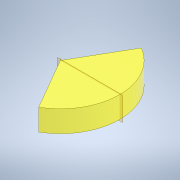
# Autodesk Inventor part: largeCap
Saved by Autodesk Inventor 2021.1 (Build 251245000, 245)
## iProperties
Created: 2020-09-25
Part Number: largeCap
Material: PC/ABS Plastic
Document SubType Name: Modeling
Designer: robst
Density: 0.357273 g/cm^3
Appearance: Smooth - Yellow
Author: robst
Autodesk Inventor part; units mm, degrees
ref_plane "XZ Plane" through (0, 0, 0) normal (0, 1, 0) x (-1, 0, 0)
sketch "Sketch1" plane through (0, 0, 0) normal (0, 0, 1) x (1, 0, 0)
  line L0 (0, 0) -> (122.2375, 0)
  line L1 (122.2375, 0) -> (122.2375, -44.45)
  line L2 (122.2375, -44.45) -> (115.8875, -44.45)
  line L3 (115.8875, -44.45) -> (115.8875, -6.35)
  line L4 (115.8875, -6.35) -> (0, -6.35)
  line L5 (0, -6.35) -> (0, 0)
  dimension "d2" = 6.35
  dimension "d3" = 6.35
  dimension "d4" = 115.8875
  dimension "d5" = 38.1
  constraints: 12 end point, 4 perpendicular, 1 horizontal, 1 parallel
  measures "d2" distance between parallel lines of L4 L0
  measures "d3" distance between parallel lines of L1 L3
  measures "d4" distance from line of L3 L0.start
  measures "d5" distance from line of L2.end L4
revolve "Revolution1" add sketch "Sketch1" angle 120 mid plane about axis through (0, -6.35, 0) along (0, 1, 0)
ref_plane "Work Plane1" through (57.9438, -44.45, -100.3615) normal (1, 0, 0) x (0, 1, 0)
sketch "Sketch7" plane through (57.9438, -44.45, -100.3615) normal (1, 0, 0) x (0, 1, 0)
  line L0 (38.1, 0) -> (38.1, 100.3615) projected
  line L1 (44.45, 100.3615) -> (38.1, 100.3615) projected
  line L2 (44.45, 100.3615) -> (44.45, -5.4993) projected
  line L3 (44.45, -5.4993) -> (0, -5.4993) projected
  line L4 (0, -5.4993) -> (0, 0) projected
  line L5 (0, 0) -> (38.1, 0) projected
  line L6 (38.1, 0) -> (38.1, 200.723) projected
  line L7 (38.1, 100.3615) -> (38.1, 200.723) projected
  line L8 (38.1, 200.723) -> (0, 200.723) projected
  line L9 (0, 200.723) -> (0, 206.2223) projected
  line L10 (0, 206.2223) -> (44.45, 206.2223) projected
  line L11 (44.45, 206.2223) -> (44.45, 100.3615) projected
  line L12 (44.45, 100.3615) -> (38.1, 100.3615) projected
  line L13 (19.05, 0) -> (19.05, 200.723) construction
  line L14 (15.24, 56.8306) -> (15.24, 52.4154)
  line L15 (15.24, 52.4154) -> (22.86, 52.4154)
  line L16 (22.86, 52.4154) -> (22.86, 53.4281)
  line L17 (22.86, 53.4281) -> (16.1416, 53.4281)
  line L18 (16.1416, 53.4281) -> (16.1416, 56.8306)
  line L19 (16.1416, 56.8306) -> (15.24, 56.8306)
  spline S0 degree 2 poles (15.8452, 60.7394) (15.7587, 60.622) (15.45, 60.2268) (15.3573, 60.0416) knots 0 0 0 1 2 2 2
  spline S1 degree 2 poles (15.3573, 60.0416) (15.2215, 59.7884) (15.0794, 59.3129) (15.0794, 58.8807) knots 0 0 0 1 2 2 2
  spline S2 degree 2 poles (15.0794, 58.8807) (15.0794, 58.5287) (15.345, 57.8927) (15.5858, 57.6518) knots 0 0 0 1 2 2 2
  spline S3 degree 2 poles (15.5858, 57.6518) (15.8205, 57.4234) (16.5121, 57.1455) (16.8949, 57.1455) knots 0 0 0 1 2 2 2
  spline S4 degree 2 poles (16.8949, 57.1455) (17.4877, 57.1455) (18.3275, 57.6457) (18.5683, 58.1891) knots 0 0 0 1 2 2 2
  spline S5 degree 2 poles (18.5683, 58.1891) (18.7906, 58.6707) (18.9574, 59.9798) (19.0006, 60.7394) knots 0 0 0 1 2 2 2
  line L20 (19.0006, 60.7394) -> (19.1859, 60.7394)
  spline S6 degree 2 poles (19.1859, 60.7394) (19.5193, 60.7394) (19.933, 60.5356) (20.0504, 60.3503) knots 0 0 0 1 2 2 2
  spline S7 degree 2 poles (20.0504, 60.3503) (20.1677, 60.1651) (20.2418, 59.634) (20.2418, 59.35) knots 0 0 0 1 2 2 2
  spline S8 degree 2 poles (20.2418, 59.35) (20.2418, 59.0165) (20.0442, 58.115) (19.8528, 57.6642) knots 0 0 0 1 2 2 2
  line L21 (19.8528, 57.6642) -> (19.8528, 57.6086)
  line L22 (19.8528, 57.6086) -> (20.8346, 57.6086)
  spline S9 degree 2 poles (20.8346, 57.6086) (20.9087, 57.8741) (21.0939, 58.8683) (21.0939, 59.3562) knots 0 0 0 1 2 2 2
  spline S10 degree 2 poles (21.0939, 59.3562) (21.0939, 59.949) (20.9087, 60.7579) (20.6679, 61.079) knots 0 0 0 1 2 2 2
  spline S11 degree 2 poles (20.6679, 61.079) (20.4332, 61.3939) (19.686, 61.7027) (19.1488, 61.7027) knots 0 0 0 1 2 2 2
  line L23 (19.1488, 61.7027) -> (15.24, 61.7027)
  line L24 (15.24, 61.7027) -> (15.24, 60.7394)
  line L25 (15.24, 60.7394) -> (15.8452, 60.7394)
  line L26 (16.6479, 60.7394) -> (18.2349, 60.7394)
  spline S12 degree 2 poles (18.2349, 60.7394) (18.204, 60.3936) (18.099, 59.35) (18.0002, 59.0227) knots 0 0 0 1 2 2 2
  spline S13 degree 2 poles (18.0002, 59.0227) (17.8829, 58.6399) (17.3951, 58.1397) (16.9628, 58.1397) knots 0 0 0 1 2 2 2
  spline S14 degree 2 poles (16.9628, 58.1397) (16.4688, 58.1397) (15.9687, 58.6954) (15.9687, 59.2265) knots 0 0 0 1 2 2 2
  spline S15 degree 2 poles (15.9687, 59.2265) (15.9687, 59.6773) (16.3577, 60.4183) (16.6479, 60.7394) knots 0 0 0 1 2 2 2
  line L27 (19.9269, 66.087) -> (19.9269, 66.0376)
  spline S16 degree 2 poles (19.9269, 66.0376) (19.9577, 65.9264) (19.9701, 65.6856) (19.9701, 65.5188) knots 0 0 0 1 2 2 2
  spline S17 degree 2 poles (19.9701, 65.5188) (19.9701, 65.1298) (19.6305, 64.3641) (19.297, 64.0183) knots 0 0 0 1 2 2 2
  line L28 (19.297, 64.0183) -> (15.24, 64.0183)
  line L29 (15.24, 64.0183) -> (15.24, 63.055)
  line L30 (15.24, 63.055) -> (20.9581, 63.055)
  line L31 (20.9581, 63.055) -> (20.9581, 64.0183)
  line L32 (20.9581, 64.0183) -> (20.1059, 64.0183)
  spline S18 degree 2 poles (20.1059, 64.0183) (20.5752, 64.5432) (20.9581, 65.3274) (20.9581, 65.6979) knots 0 0 0 1 2 2 2
  spline S19 degree 2 poles (20.9581, 65.6979) (20.9581, 65.8461) (20.9457, 65.9943) (20.9272, 66.087) knots 0 0 0 1 2 2 2
  line L33 (20.9272, 66.087) -> (19.9269, 66.087)
  spline S20 degree 2 poles (14.3261, 67.0379) (14.2829, 67.1367) (14.147, 67.5134) (14.0914, 67.7542) knots 0 0 0 1 2 2 2
  spline S21 degree 2 poles (14.0914, 67.7542) (14.0235, 68.0197) (13.9432, 68.4705) (13.9432, 68.736) knots 0 0 0 1 2 2 2
  spline S22 degree 2 poles (13.9432, 68.736) (13.9432, 69.1806) (14.1779, 69.7982) (14.3878, 69.9711) knots 0 0 0 1 2 2 2
  spline S23 degree 2 poles (14.3878, 69.9711) (14.5978, 70.1378) (15.1474, 70.2675) (15.4994, 70.2675) knots 0 0 0 1 2 2 2
  line L34 (15.4994, 70.2675) -> (15.9995, 70.2675)
  spline S24 degree 2 poles (15.9995, 70.2675) (15.6599, 69.8784) (15.3388, 69.1312) (15.3388, 68.5693) knots 0 0 0 1 2 2 2
  spline S25 degree 2 poles (15.3388, 68.5693) (15.3388, 67.5937) (16.7899, 66.4389) (18.1546, 66.4389) knots 0 0 0 1 2 2 2
  spline S26 degree 2 poles (18.1546, 66.4389) (18.8647, 66.4389) (19.9639, 66.8403) (20.3529, 67.1738) knots 0 0 0 1 2 2 2
  spline S27 degree 2 poles (20.3529, 67.1738) (20.7173, 67.4949) (21.1186, 68.3779) (21.1186, 68.8472) knots 0 0 0 1 2 2 2
  spline S28 degree 2 poles (21.1186, 68.8472) (21.1186, 69.2918) (20.9087, 69.9402) (20.7173, 70.2675) knots 0 0 0 1 2 2 2
  line L35 (20.7173, 70.2675) -> (20.9581, 70.323)
  line L36 (20.9581, 70.323) -> (20.9581, 71.2308)
  line L37 (20.9581, 71.2308) -> (15.8946, 71.2308)
  spline S29 degree 2 poles (15.8946, 71.2308) (14.4372, 71.2308) (13.0787, 69.9649) (13.0787, 68.6619) knots 0 0 0 1 2 2 2
  spline S30 degree 2 poles (13.0787, 68.6619) (13.0787, 68.242) (13.2146, 67.3652) (13.3257, 66.9885) knots 0 0 0 1 2 2 2
  line L38 (13.3257, 66.9885) -> (14.3261, 66.9885)
  line L39 (14.3261, 66.9885) -> (14.3261, 67.0379)
  line L40 (16.7899, 70.2675) -> (19.933, 70.2675)
  spline S31 degree 2 poles (19.933, 70.2675) (20.1059, 69.9093) (20.2541, 69.3041) (20.2541, 69.0016) knots 0 0 0 1 2 2 2
  spline S32 degree 2 poles (20.2541, 69.0016) (20.2541, 68.2729) (19.1797, 67.4331) (18.1731, 67.4331) knots 0 0 0 1 2 2 2
  spline S33 degree 2 poles (18.1731, 67.4331) (17.2222, 67.4331) (16.228, 68.0691) (16.228, 68.7854) knots 0 0 0 1 2 2 2
  spline S34 degree 2 poles (16.228, 68.7854) (16.228, 69.1621) (16.5244, 69.9525) (16.7899, 70.2675) knots 0 0 0 1 2 2 2
  spline S35 degree 2 poles (15.1103, 75.1087) (15.1103, 73.7378) (16.6479, 72.2311) (18.0682, 72.2311) knots 0 0 0 1 2 2 2
  spline S36 degree 2 poles (18.0682, 72.2311) (19.4637, 72.2311) (21.1186, 73.6946) (21.1186, 74.874) knots 0 0 0 1 2 2 2
  spline S37 degree 2 poles (21.1186, 74.874) (21.1186, 75.4051) (20.8099, 76.2264) (20.4826, 76.5289) knots 0 0 0 1 2 2 2
  spline S38 degree 2 poles (20.4826, 76.5289) (20.1553, 76.8377) (19.2106, 77.165) (18.5251, 77.165) knots 0 0 0 1 2 2 2
  line L41 (18.5251, 77.165) -> (18.0002, 77.165)
  line L42 (18.0002, 77.165) -> (18.0002, 73.2068)
  spline S39 degree 2 poles (18.0002, 73.2068) (17.0061, 73.2068) (15.9501, 74.2071) (15.9501, 75.0963) knots 0 0 0 1 2 2 2
  spline S40 degree 2 poles (15.9501, 75.0963) (15.9501, 75.4113) (16.0922, 76.0226) (16.2033, 76.2696) knots 0 0 0 1 2 2 2
  spline S41 degree 2 poles (16.2033, 76.2696) (16.3268, 76.5289) (16.5429, 76.8871) (16.6417, 77.0044) knots 0 0 0 1 2 2 2
  line L43 (16.6417, 77.0044) -> (16.6417, 77.06)
  line L44 (16.6417, 77.06) -> (15.592, 77.06)
  spline S42 degree 2 poles (15.592, 77.06) (15.5241, 76.8933) (15.3265, 76.3869) (15.2709, 76.1893) knots 0 0 0 1 2 2 2
  spline S43 degree 2 poles (15.2709, 76.1893) (15.1906, 75.9114) (15.1103, 75.4545) (15.1103, 75.1087) knots 0 0 0 1 2 2 2
  spline S44 degree 2 poles (18.7351, 76.2264) (19.1241, 76.214) (19.6922, 76.0535) (19.8836, 75.8991) knots 0 0 0 1 2 2 2
  spline S45 degree 2 poles (19.8836, 75.8991) (20.0998, 75.7324) (20.3282, 75.2075) (20.3282, 74.8185) knots 0 0 0 1 2 2 2
  spline S46 degree 2 poles (20.3282, 74.8185) (20.3282, 74.4356) (20.0998, 73.8984) (19.8775, 73.6761) knots 0 0 0 1 2 2 2
  spline S47 degree 2 poles (19.8775, 73.6761) (19.649, 73.46) (19.0994, 73.2377) (18.7351, 73.2068) knots 0 0 0 1 2 2 2
  line L45 (18.7351, 73.2068) -> (18.7351, 76.2264)
  spline S48 degree 2 poles (15.1041, 84.4639) (15.1041, 83.7229) (15.6043, 82.4693) (16.1045, 82.0124) knots 0 0 0 1 2 2 2
  spline S49 degree 2 poles (16.1045, 82.0124) (16.5985, 81.5554) (18.0805, 81.0553) (19.0438, 81.0553) knots 0 0 0 1 2 2 2
  spline S50 degree 2 poles (19.0438, 81.0553) (20.001, 81.0553) (21.4212, 81.5431) (21.9461, 82.0062) knots 0 0 0 1 2 2 2
  spline S51 degree 2 poles (21.9461, 82.0062) (22.4586, 82.4632) (22.9959, 83.7105) (22.9959, 84.4824) knots 0 0 0 1 2 2 2
  spline S52 degree 2 poles (22.9959, 84.4824) (22.9959, 84.8653) (22.8847, 85.5383) (22.7982, 85.8224) knots 0 0 0 1 2 2 2
  spline S53 degree 2 poles (22.7982, 85.8224) (22.718, 86.0694) (22.4895, 86.5819) (22.3536, 86.8351) knots 0 0 0 1 2 2 2
  line L46 (22.3536, 86.8351) -> (21.131, 86.8351)
  line L47 (21.131, 86.8351) -> (21.131, 86.7548)
  spline S54 degree 2 poles (21.131, 86.7548) (21.2545, 86.619) (21.6003, 86.1991) (21.767, 85.8965) knots 0 0 0 1 2 2 2
  spline S55 degree 2 poles (21.767, 85.8965) (21.9276, 85.6063) (22.1313, 84.9208) (22.1313, 84.4762) knots 0 0 0 1 2 2 2
  spline S56 degree 2 poles (22.1313, 84.4762) (22.1313, 83.9884) (21.73, 83.1177) (21.3471, 82.7904) knots 0 0 0 1 2 2 2
  spline S57 degree 2 poles (21.3471, 82.7904) (20.9581, 82.4693) (19.7787, 82.1112) (19.0438, 82.1112) knots 0 0 0 1 2 2 2
  spline S58 degree 2 poles (19.0438, 82.1112) (18.2596, 82.1112) (17.1296, 82.4879) (16.7405, 82.8151) knots 0 0 0 1 2 2 2
  spline S59 degree 2 poles (16.7405, 82.8151) (16.3639, 83.1362) (15.981, 83.9946) (15.981, 84.4762) knots 0 0 0 1 2 2 2
  spline S60 degree 2 poles (15.981, 84.4762) (15.981, 84.9147) (16.1971, 85.6618) (16.3577, 85.9521) knots 0 0 0 1 2 2 2
  spline S61 degree 2 poles (16.3577, 85.9521) (16.5182, 86.2299) (16.8517, 86.6437) (16.969, 86.761) knots 0 0 0 1 2 2 2
  line L48 (16.969, 86.761) -> (16.969, 86.8351)
  line L49 (16.969, 86.8351) -> (15.7587, 86.8351)
  spline S62 degree 2 poles (15.7587, 86.8351) (15.6414, 86.5819) (15.4253, 86.1373) (15.3265, 85.8224) knots 0 0 0 1 2 2 2
  spline S63 degree 2 poles (15.3265, 85.8224) (15.2153, 85.4889) (15.1041, 84.9208) (15.1041, 84.4639) knots 0 0 0 1 2 2 2
  spline S64 degree 2 poles (15.8452, 90.8921) (15.7587, 90.7748) (15.45, 90.3796) (15.3573, 90.1943) knots 0 0 0 1 2 2 2
  spline S65 degree 2 poles (15.3573, 90.1943) (15.2215, 89.9411) (15.0794, 89.4657) (15.0794, 89.0334) knots 0 0 0 1 2 2 2
  spline S66 degree 2 poles (15.0794, 89.0334) (15.0794, 88.6814) (15.345, 88.0454) (15.5858, 87.8046) knots 0 0 0 1 2 2 2
  spline S67 degree 2 poles (15.5858, 87.8046) (15.8205, 87.5761) (16.5121, 87.2982) (16.8949, 87.2982) knots 0 0 0 1 2 2 2
  spline S68 degree 2 poles (16.8949, 87.2982) (17.4877, 87.2982) (18.3275, 87.7984) (18.5683, 88.3418) knots 0 0 0 1 2 2 2
  spline S69 degree 2 poles (18.5683, 88.3418) (18.7906, 88.8235) (18.9574, 90.1326) (19.0006, 90.8921) knots 0 0 0 1 2 2 2
  line L50 (19.0006, 90.8921) -> (19.1859, 90.8921)
  spline S70 degree 2 poles (19.1859, 90.8921) (19.5193, 90.8921) (19.933, 90.6883) (20.0504, 90.5031) knots 0 0 0 1 2 2 2
  spline S71 degree 2 poles (20.0504, 90.5031) (20.1677, 90.3178) (20.2418, 89.7868) (20.2418, 89.5027) knots 0 0 0 1 2 2 2
  spline S72 degree 2 poles (20.2418, 89.5027) (20.2418, 89.1693) (20.0442, 88.2677) (19.8528, 87.8169) knots 0 0 0 1 2 2 2
  line L51 (19.8528, 87.8169) -> (19.8528, 87.7613)
  line L52 (19.8528, 87.7613) -> (20.8346, 87.7613)
  spline S73 degree 2 poles (20.8346, 87.7613) (20.9087, 88.0269) (21.0939, 89.0211) (21.0939, 89.5089) knots 0 0 0 1 2 2 2
  spline S74 degree 2 poles (21.0939, 89.5089) (21.0939, 90.1017) (20.9087, 90.9106) (20.6679, 91.2317) knots 0 0 0 1 2 2 2
  spline S75 degree 2 poles (20.6679, 91.2317) (20.4332, 91.5466) (19.686, 91.8554) (19.1488, 91.8554) knots 0 0 0 1 2 2 2
  line L53 (19.1488, 91.8554) -> (15.24, 91.8554)
  line L54 (15.24, 91.8554) -> (15.24, 90.8921)
  line L55 (15.24, 90.8921) -> (15.8452, 90.8921)
  line L56 (16.6479, 90.8921) -> (18.2349, 90.8921)
  spline S76 degree 2 poles (18.2349, 90.8921) (18.204, 90.5463) (18.099, 89.5027) (18.0002, 89.1754) knots 0 0 0 1 2 2 2
  spline S77 degree 2 poles (18.0002, 89.1754) (17.8829, 88.7926) (17.3951, 88.2924) (16.9628, 88.2924) knots 0 0 0 1 2 2 2
  spline S78 degree 2 poles (16.9628, 88.2924) (16.4688, 88.2924) (15.9687, 88.8482) (15.9687, 89.3792) knots 0 0 0 1 2 2 2
  spline S79 degree 2 poles (15.9687, 89.3792) (15.9687, 89.83) (16.3577, 90.571) (16.6479, 90.8921) knots 0 0 0 1 2 2 2
  spline S80 degree 2 poles (18.2534, 97.9996) (16.8208, 97.9996) (15.1288, 96.6349) (15.1288, 95.5913) knots 0 0 0 1 2 2 2
  spline S81 degree 2 poles (15.1288, 95.5913) (15.1288, 95.1652) (15.3265, 94.5107) (15.5302, 94.171) knots 0 0 0 1 2 2 2
  line L57 (15.5302, 94.171) -> (13.1343, 94.171)
  line L58 (13.1343, 94.171) -> (13.1343, 93.2077)
  line L59 (13.1343, 93.2077) -> (20.9581, 93.2077)
  line L60 (20.9581, 93.2077) -> (20.9581, 94.171)
  line L61 (20.9581, 94.171) -> (20.3591, 94.171)
  spline S82 degree 2 poles (20.3591, 94.171) (20.6864, 94.5292) (21.1186, 95.406) (21.1186, 95.9186) knots 0 0 0 1 2 2 2
  spline S83 degree 2 poles (21.1186, 95.9186) (21.1186, 96.9004) (19.5625, 97.9996) (18.2534, 97.9996) knots 0 0 0 1 2 2 2
  spline S84 degree 2 poles (18.1423, 97.0054) (19.1241, 97.0054) (20.2047, 96.3817) (20.2047, 95.6839) knots 0 0 0 1 2 2 2
  spline S85 degree 2 poles (20.2047, 95.6839) (20.2047, 95.2764) (19.8404, 94.5107) (19.5564, 94.171) knots 0 0 0 1 2 2 2
  line L62 (19.5564, 94.171) -> (16.3083, 94.171)
  spline S86 degree 2 poles (16.3083, 94.171) (16.1292, 94.5477) (15.9934, 95.0849) (15.9934, 95.4307) knots 0 0 0 1 2 2 2
  spline S87 degree 2 poles (15.9934, 95.4307) (15.9934, 96.1779) (17.0925, 97.0054) (18.1423, 97.0054) knots 0 0 0 1 2 2 2
  spline S88 degree 2 poles (15.0918, 105.5393) (15.0918, 104.7304) (15.5858, 103.3904) (16.086, 102.9087) knots 0 0 0 1 2 2 2
  spline S89 degree 2 poles (16.086, 102.9087) (16.5923, 102.4271) (18.0867, 101.9145) (19.0562, 101.9145) knots 0 0 0 1 2 2 2
  spline S90 degree 2 poles (19.0562, 101.9145) (19.9763, 101.9145) (21.4336, 102.4332) (21.9523, 102.9149) knots 0 0 0 1 2 2 2
  spline S91 degree 2 poles (21.9523, 102.9149) (22.4524, 103.378) (22.9959, 104.7365) (22.9959, 105.5455) knots 0 0 0 1 2 2 2
  spline S92 degree 2 poles (22.9959, 105.5455) (22.9959, 105.9345) (22.8847, 106.6384) (22.7859, 106.9595) knots 0 0 0 1 2 2 2
  spline S93 degree 2 poles (22.7859, 106.9595) (22.7118, 107.2189) (22.4401, 107.8488) (22.3413, 108.0402) knots 0 0 0 1 2 2 2
  line L63 (22.3413, 108.0402) -> (21.1186, 108.0402)
  line L64 (21.1186, 108.0402) -> (21.1186, 107.9537)
  spline S94 degree 2 poles (21.1186, 107.9537) (21.2854, 107.7623) (21.5879, 107.3609) (21.7608, 106.9904) knots 0 0 0 1 2 2 2
  spline S95 degree 2 poles (21.7608, 106.9904) (21.9152, 106.6817) (22.119, 105.8851) (22.119, 105.4281) knots 0 0 0 1 2 2 2
  spline S96 degree 2 poles (22.119, 105.4281) (22.119, 104.329) (20.4641, 102.9705) (19.0871, 102.9705) knots 0 0 0 1 2 2 2
  spline S97 degree 2 poles (19.0871, 102.9705) (18.3213, 102.9705) (17.1728, 103.3286) (16.7776, 103.6683) knots 0 0 0 1 2 2 2
  spline S98 degree 2 poles (16.7776, 103.6683) (16.3824, 103.9955) (15.9687, 104.9218) (15.9687, 105.5022) knots 0 0 0 1 2 2 2
  spline S99 degree 2 poles (15.9687, 105.5022) (15.9687, 105.9283) (16.0922, 106.7805) (16.2157, 107.0707) knots 0 0 0 1 2 2 2
  line L65 (16.2157, 107.0707) -> (18.1855, 107.0707)
  line L66 (18.1855, 107.0707) -> (18.1855, 105.3046)
  line L67 (18.1855, 105.3046) -> (19.0747, 105.3046)
  line L68 (19.0747, 105.3046) -> (19.0747, 108.0711)
  line L69 (19.0747, 108.0711) -> (15.7464, 108.0711)
  spline S100 degree 2 poles (15.7464, 108.0711) (15.6599, 107.8796) (15.3944, 107.2251) (15.3141, 106.9472) knots 0 0 0 1 2 2 2
  spline S101 degree 2 poles (15.3141, 106.9472) (15.2029, 106.5705) (15.0918, 105.9654) (15.0918, 105.5393) knots 0 0 0 1 2 2 2
  line L70 (15.24, 110.2508) -> (15.24, 109.2875)
  line L71 (15.24, 109.2875) -> (23.1996, 109.2875)
  line L72 (23.1996, 109.2875) -> (23.1996, 110.2508)
  line L73 (23.1996, 110.2508) -> (15.24, 110.2508)
  line L74 (15.24, 116.111) -> (15.24, 115.1477)
  line L75 (15.24, 115.1477) -> (15.8699, 115.1477)
  spline S102 degree 2 poles (15.8699, 115.1477) (15.4808, 114.703) (15.0794, 113.9065) (15.0794, 113.4125) knots 0 0 0 1 2 2 2
  spline S103 degree 2 poles (15.0794, 113.4125) (15.0794, 113.042) (15.3265, 112.3812) (15.592, 112.1404) knots 0 0 0 1 2 2 2
  spline S104 degree 2 poles (15.592, 112.1404) (15.8575, 111.8934) (16.6664, 111.6217) (17.2469, 111.6217) knots 0 0 0 1 2 2 2
  line L76 (17.2469, 111.6217) -> (20.9581, 111.6217)
  line L77 (20.9581, 111.6217) -> (20.9581, 112.585)
  line L78 (20.9581, 112.585) -> (17.6977, 112.585)
  spline S105 degree 2 poles (17.6977, 112.585) (17.2407, 112.585) (16.6417, 112.6529) (16.4194, 112.7703) knots 0 0 0 1 2 2 2
  spline S106 degree 2 poles (16.4194, 112.7703) (16.1971, 112.8876) (15.9934, 113.289) (15.9934, 113.6656) knots 0 0 0 1 2 2 2
  spline S107 degree 2 poles (15.9934, 113.6656) (15.9934, 114.0176) (16.3947, 114.8142) (16.685, 115.1477) knots 0 0 0 1 2 2 2
  line L79 (16.685, 115.1477) -> (20.9581, 115.1477)
  line L80 (20.9581, 115.1477) -> (20.9581, 116.111)
  line L81 (20.9581, 116.111) -> (15.24, 116.111)
  spline S108 degree 2 poles (15.1103, 119.9889) (15.1103, 118.618) (16.6479, 117.1113) (18.0682, 117.1113) knots 0 0 0 1 2 2 2
  spline S109 degree 2 poles (18.0682, 117.1113) (19.4637, 117.1113) (21.1186, 118.5748) (21.1186, 119.7542) knots 0 0 0 1 2 2 2
  spline S110 degree 2 poles (21.1186, 119.7542) (21.1186, 120.2853) (20.8099, 121.1066) (20.4826, 121.4091) knots 0 0 0 1 2 2 2
  spline S111 degree 2 poles (20.4826, 121.4091) (20.1553, 121.7179) (19.2106, 122.0452) (18.5251, 122.0452) knots 0 0 0 1 2 2 2
  line L82 (18.5251, 122.0452) -> (18.0002, 122.0452)
  line L83 (18.0002, 122.0452) -> (18.0002, 118.087)
  spline S112 degree 2 poles (18.0002, 118.087) (17.0061, 118.087) (15.9501, 119.0873) (15.9501, 119.9765) knots 0 0 0 1 2 2 2
  spline S113 degree 2 poles (15.9501, 119.9765) (15.9501, 120.2915) (16.0922, 120.9028) (16.2033, 121.1498) knots 0 0 0 1 2 2 2
  spline S114 degree 2 poles (16.2033, 121.1498) (16.3268, 121.4091) (16.5429, 121.7673) (16.6417, 121.8846) knots 0 0 0 1 2 2 2
  line L84 (16.6417, 121.8846) -> (16.6417, 121.9402)
  line L85 (16.6417, 121.9402) -> (15.592, 121.9402)
  spline S115 degree 2 poles (15.592, 121.9402) (15.5241, 121.7735) (15.3265, 121.2671) (15.2709, 121.0695) knots 0 0 0 1 2 2 2
  spline S116 degree 2 poles (15.2709, 121.0695) (15.1906, 120.7916) (15.1103, 120.3347) (15.1103, 119.9889) knots 0 0 0 1 2 2 2
  spline S117 degree 2 poles (18.7351, 121.1066) (19.1241, 121.0942) (19.6922, 120.9337) (19.8836, 120.7793) knots 0 0 0 1 2 2 2
  spline S118 degree 2 poles (19.8836, 120.7793) (20.0998, 120.6126) (20.3282, 120.0877) (20.3282, 119.6987) knots 0 0 0 1 2 2 2
  spline S119 degree 2 poles (20.3282, 119.6987) (20.3282, 119.3158) (20.0998, 118.7786) (19.8775, 118.5563) knots 0 0 0 1 2 2 2
  spline S120 degree 2 poles (19.8775, 118.5563) (19.649, 118.3401) (19.0994, 118.1178) (18.7351, 118.087) knots 0 0 0 1 2 2 2
  line L86 (18.7351, 118.087) -> (18.7351, 121.1066)
  line L87 (15.24, 127.4175) -> (15.24, 126.4542)
  line L88 (15.24, 126.4542) -> (15.8205, 126.4542)
  spline S121 degree 2 poles (15.8205, 126.4542) (15.6352, 126.2318) (15.3882, 125.9046) (15.2832, 125.6823) knots 0 0 0 1 2 2 2
  spline S122 degree 2 poles (15.2832, 125.6823) (15.1844, 125.4785) (15.0794, 125.0401) (15.0794, 124.7498) knots 0 0 0 1 2 2 2
  spline S123 degree 2 poles (15.0794, 124.7498) (15.0794, 124.2805) (15.4685, 123.4901) (15.8452, 123.2123) knots 0 0 0 1 2 2 2
  spline S124 degree 2 poles (15.8452, 123.2123) (16.2218, 122.9344) (17.3333, 122.6256) (18.0558, 122.6256) knots 0 0 0 1 2 2 2
  spline S125 degree 2 poles (18.0558, 122.6256) (18.8092, 122.6256) (19.9083, 123.0147) (20.3221, 123.3543) knots 0 0 0 1 2 2 2
  spline S126 degree 2 poles (20.3221, 123.3543) (20.6926, 123.6692) (21.1186, 124.5522) (21.1186, 125.0401) knots 0 0 0 1 2 2 2
  spline S127 degree 2 poles (21.1186, 125.0401) (21.1186, 125.4661) (20.9272, 126.1022) (20.7296, 126.4542) knots 0 0 0 1 2 2 2
  line L89 (20.7296, 126.4542) -> (23.1996, 126.4542)
  line L90 (23.1996, 126.4542) -> (23.1996, 127.4175)
  line L91 (23.1996, 127.4175) -> (15.24, 127.4175)
  line L92 (16.6294, 126.4542) -> (19.933, 126.4542)
  spline S128 degree 2 poles (19.933, 126.4542) (20.1059, 126.096) (20.2356, 125.5279) (20.2356, 125.2006) knots 0 0 0 1 2 2 2
  spline S129 degree 2 poles (20.2356, 125.2006) (20.2356, 124.4596) (19.1241, 123.6198) (18.0743, 123.6198) knots 0 0 0 1 2 2 2
  spline S130 degree 2 poles (18.0743, 123.6198) (17.0616, 123.6198) (15.9934, 124.262) (15.9934, 124.9721) knots 0 0 0 1 2 2 2
  spline S131 degree 2 poles (15.9934, 124.9721) (15.9934, 125.3488) (16.3392, 126.1145) (16.6294, 126.4542) knots 0 0 0 1 2 2 2
  line L93 (22.86, 137.6865) -> (15.24, 135.0622)
  line L94 (15.24, 135.0622) -> (15.24, 133.9692)
  line L95 (15.24, 133.9692) -> (22.86, 131.3448)
  line L96 (22.86, 131.3448) -> (22.86, 132.4316)
  line L97 (22.86, 132.4316) -> (16.5306, 134.5435)
  line L98 (16.5306, 134.5435) -> (22.86, 136.6553)
  line L99 (22.86, 136.6553) -> (22.86, 137.6865)
  spline S132 degree 2 poles (19.05, 143.028) (16.9999, 143.028) (15.0794, 141.8362) (15.0794, 140.595) knots 0 0 0 1 2 2 2
  spline S133 degree 2 poles (15.0794, 140.595) (15.0794, 139.3353) (17.0369, 138.1559) (19.0438, 138.1559) knots 0 0 0 1 2 2 2
  spline S134 degree 2 poles (19.0438, 138.1559) (21.1063, 138.1559) (23.0144, 139.3476) (23.0144, 140.595) knots 0 0 0 1 2 2 2
  spline S135 degree 2 poles (23.0144, 140.595) (23.0144, 141.8485) (21.0384, 143.028) (19.05, 143.028) knots 0 0 0 1 2 2 2
  spline S136 degree 2 poles (16.7282, 141.7189) (17.1049, 141.8671) (18.2658, 141.9906) (19.05, 141.9906) knots 0 0 0 1 2 2 2
  spline S137 degree 2 poles (19.05, 141.9906) (19.8342, 141.9906) (20.989, 141.8671) (21.378, 141.7127) knots 0 0 0 1 2 2 2
  spline S138 degree 2 poles (21.378, 141.7127) (21.767, 141.5583) (22.1684, 141.0211) (22.1684, 140.595) knots 0 0 0 1 2 2 2
  spline S139 degree 2 poles (22.1684, 140.595) (22.1684, 140.1689) (21.767, 139.6193) (21.3656, 139.4588) knots 0 0 0 1 2 2 2
  spline S140 degree 2 poles (21.3656, 139.4588) (20.9766, 139.3044) (19.791, 139.1933) (19.0438, 139.1933) knots 0 0 0 1 2 2 2
  spline S141 degree 2 poles (19.0438, 139.1933) (18.2411, 139.1933) (17.1666, 139.2921) (16.7467, 139.4526) knots 0 0 0 1 2 2 2
  spline S142 degree 2 poles (16.7467, 139.4526) (16.3515, 139.6008) (15.9254, 140.1504) (15.9254, 140.595) knots 0 0 0 1 2 2 2
  spline S143 degree 2 poles (15.9254, 140.595) (15.9254, 141.0149) (16.3268, 141.5645) (16.7282, 141.7189) knots 0 0 0 1 2 2 2
  line L100 (15.24, 148.32) -> (15.24, 144.6026)
  line L101 (15.24, 144.6026) -> (16.0181, 144.6026)
  line L102 (16.0181, 144.6026) -> (16.0181, 145.9858)
  line L103 (16.0181, 145.9858) -> (21.1248, 145.9858)
  line L104 (21.1248, 145.9858) -> (21.1248, 144.6026)
  line L105 (21.1248, 144.6026) -> (21.8226, 144.6026)
  spline S144 degree 2 poles (21.8226, 144.6026) (21.8226, 145.3868) (22.2672, 146.1278) (22.8847, 146.1772) knots 0 0 0 1 2 2 2
  line L106 (22.8847, 146.1772) -> (22.8847, 146.9676)
  line L107 (22.8847, 146.9676) -> (16.0181, 146.9676)
  line L108 (16.0181, 146.9676) -> (16.0181, 148.32)
  line L109 (16.0181, 148.32) -> (15.24, 148.32)
  constraints: 2 end point, 2 midpoint, 1 vertical
emboss "Emboss1" sketch "Sketch7" operation cut depth 1.27 direction (-1, 0, 0) wrap yes faces at (88.775, -19.05, 74.491) contours L19 L18 L17 L16 L15 L14 | L25 L24 L23 S11 S10 S9 L22 L21 S8 S7 S6 L20 S5 S4 S3 S2 S1 S0 | L33 S19 S18 L32 L31 L30 L29 L28 S17 S16 L27 | L39 L38 S30 S29 L37 L36 L35 S28 S27 S26 S25 S24 L34 S23 S22 S21 S20 | S43 S42 L44 L43 S41 S40 S39 L42 L41 S38 S37 S36 S35 | S63 S62 L49 L48 S61 S60 S59 S58 S57 S56 S55 S54 L47 L46 S53 S52 S51 S50 S49 S48 | L55 L54 L53 S75 S74 S73 L52 L51 S72 S71 S70 L50 S69 S68 S67 S66 S65 S64 | S83 S82 L61 L60 L59 L58 L57 S81 S80 | S101 S100 L69 L68 L67 L66 L65 S99 S98 S97 S96 S95 S94 L64 L63 S93 S92 S91 S90 S89 S88 | L73 L72 L71 L70 | L81 L80 L79 S107 S106 S105 L78 L77 L76 S104 S103 S102 L75 L74 | S116 S115 L85 L84 S114 S113 S112 L83 L82 S111 S110 S109 S108 | L91 L90 L89 S127 S126 S125 S124 S123 S122 S121 L88 L87 | L99 L98 L97 L96 L95 L94 L93 | S135 S134 S133 S132 | L109 L108 L107 L106 S144 L105 L104 L103 L102 L101 L100
sketch "Sketch8" plane through (0, 0, 0) normal (0, 0, 1) x (1, 0, 0)
  line L0 (0, 0) -> (0, -6.35) projected
  line L1 (0, -6.35) -> (57.9438, -6.35) projected
  line L2 (115.8875, -6.35) -> (57.9438, -6.35) projected
  line L3 (69.85, -3.175) -> (63.5, -3.175)
  line L4 (69.85, -3.175) -> (76.2, -3.175)
  line L5 (63.5, -3.175) -> (63.5, -6.35)
  line L6 (76.2, -3.175) -> (76.2, -6.35)
  line L7 (76.2, -6.35) -> (63.5, -6.35)
  line L8 (0, -53.34) -> (0, 8.89) projected
  point P0 (57.15, -6.35)
  dimension "d33" = 3.175
  dimension "d34" = 69.85
  dimension "d35" = 12.7
  constraints: 10 end point, 2 collinear, 2 horizontal, 2 perpendicular, 2 point on line
  measures "d33" distance between parallel lines of L3 L2
  measures "d34" horizontal distance of L3.start L0.start
  measures "d35" distance between parallel lines of L6 L5
revolve "Revolution3" cut sketch "Sketch8" angle 120 mid plane about axis through (0, 0, 0) along (0, -1, 0)
fillet "Fillet1" radius 1.5875 2 edges at (63.5, -6.35, 0) (76.2, -6.35, 0)
equation "\"d2\" = wallThickness"
equation "\"d3\" = wallThickness"
equation "\"d4\" = insideRadius"
equation "\"d5\" = height"
equation "\"d6\" = sweepAngle"
equation "\"d33\" = glueSlotHeight"
equation "\"d34\" = glueRingRadius"
equation "\"d35\" = glueSlotWidth"
equation "\"d37\" = sweepAngle"
equation "\"insideDiameter\" = 231.775"
equation "\"insideRadius\" = 0.5 * insideDiameter"
equation "\"wallThickness\" = 6.35"
equation "\"height\" = 38.1"
equation "\"sweepAngle\" = 120deg"
equation "\"glueRingDiameter\" = 139.7"
equation "\"glueRingRadius\" = 0.5 * glueRingDiameter"
equation "\"glueSlotWidth\" = 12.7"
equation "\"glueSlotHeight\" = 3.175"
body "Solid1"
